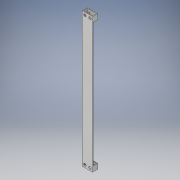
# Autodesk Inventor part: OverheadSupportBar.ver1-1111-2020
Saved by Autodesk Inventor 2018 (Build 220112000, 112)
## iProperties
Created: 2020-01-13
Part Number: OverheadSupportBar.ver1-1111-2020
Material: Generic
Document SubType Name: Modeling
Designer: JMHal
Density: 1 g/cm^3
Appearance: Default
Author: JMHal
Autodesk Inventor part; units mm, degrees
ref_plane "YZ Plane" through (0, 0, 0) normal (1, 0, 0) x (0, 1, 0)
ref_plane "XZ Plane" through (0, 0, 0) normal (0, 1, 0) x (-1, 0, 0)
ref_plane "XY Plane" through (0, 0, 0) normal (0, 0, 1) x (1, 0, 0)
sketch "Sketch1" plane through (0, 0, 0) normal (0, 1, 0) x (-1, 0, 0)
  line L0 (0, 0) -> (50.8, 0)
  line L1 (50.8, 0) -> (50.8, -25.4)
  line L2 (50.8, -25.4) -> (0, -25.4)
  line L3 (0, -25.4) -> (0, 0)
  line L4 (47.625, -3.175) -> (3.175, -3.175)
  line L5 (3.175, -3.175) -> (3.175, -22.225)
  line L6 (3.175, -22.225) -> (47.625, -22.225)
  line L7 (47.625, -22.225) -> (47.625, -3.175)
  dimension "d0" = 50.8
  dimension "d1" = 25.4
  dimension "d2" = 3.175
  constraints: 16 end point, 4 parallel, 2 perpendicular, 1 horizontal, 3 other
  measures "d0" distance of L1.end L2.end
  measures "d1" distance of L0.end L1.end
  measures "d2" distance between parallel lines of L0 L4
extrude "Extrusion1" add sketch "Sketch1" along normal blind 663.575
sketch "Sketch2" plane through (0, 0, 0) normal (1, 0, 0) x (0, 0, -1)
  line L0 (25.4, 0) -> (0, 0) projected
  line L1 (25.4, 0) -> (25.4, 663.575) projected
  line L2 (0, 663.575) -> (25.4, 663.575) projected
  line L3 (0, 0) -> (0, 663.575) projected
  line L4 (3.175, 0) -> (3.175, 663.575) projected
  line L5 (25.4, 0) -> (25.4, 663.575) projected
  line L6 (3.175, 638.175) -> (25.4, 638.175)
  line L7 (25.4, 638.175) -> (25.4, 25.4)
  line L8 (25.4, 25.4) -> (3.175, 25.4)
  line L9 (3.175, 25.4) -> (3.175, 638.175)
  dimension "d5" = 25.4
  dimension "d6" = 25.4
  constraints: 8 end point, 2 parallel, 2 point on line, 1 horizontal, 1 perpendicular
  measures "d5" distance between parallel lines of L8 L0
  measures "d6" distance between parallel lines of L2 L6
extrude "Extrusion2" cut sketch "Sketch2" against normal blind 663.575 contours L8 L4 L6 L1
sketch "Sketch3" plane through (-50.8, 0, 0) normal (0, 0, 1) x (1, 0, 0)
  line L0 (50.8, 0) -> (0, 0) projected
  line L1 (50.8, 0) -> (50.8, 663.575) projected
  line L2 (0, 663.575) -> (50.8, 663.575) projected
  line L3 (0, 0) -> (0, 663.575) projected
  line L4 (47.625, 25.4) -> (3.175, 25.4) projected
  line L5 (3.175, 0) -> (3.175, 25.4) projected
  line L6 (47.625, 0) -> (3.175, 0) projected
  line L7 (47.625, 0) -> (47.625, 25.4) projected
  line L8 (3.175, 638.175) -> (47.625, 638.175) projected
  line L9 (47.625, 638.175) -> (47.625, 663.575) projected
  line L10 (3.175, 663.575) -> (47.625, 663.575) projected
  line L11 (3.175, 638.175) -> (3.175, 663.575) projected
  point P0 (12.7, 12.7)
  point P1 (38.1, 12.7)
  point P2 (12.7, 650.875)
  point P3 (38.1, 650.875)
  dimension "d9" = 12.7
  dimension "d10" = 12.7
  dimension "d11" = 12.7
  dimension "d12" = 12.7
  dimension "d13" = 12.7
  dimension "d14" = 12.7
  dimension "d15" = 12.7
  dimension "d16" = 12.7
  measures "d9" distance from line of L3 point (12.7, 650.875)
  measures "d10" distance from line of L1 point (38.1, 650.875)
  measures "d11" distance from line of L2 point (38.1, 650.875)
  measures "d12" distance from line of L2 point (12.7, 650.875)
  measures "d13" distance from line of L0 point (12.7, 12.7)
  measures "d14" distance from line of L3 point (12.7, 12.7)
  measures "d15" distance from line of L1 point (38.1, 12.7)
  measures "d16" distance from line of L0 point (38.1, 12.7)
hole "Hole1" at (-38.1, 12.7, 0) at (-12.7, 12.7, 0) at (-38.1, 650.875, 0) at (-12.7, 650.875, 0) direction (0, 0, -1) diameter 6.35 end through all counterbore diameter 12.7 counterbore depth 6.35
body "Solid1"
